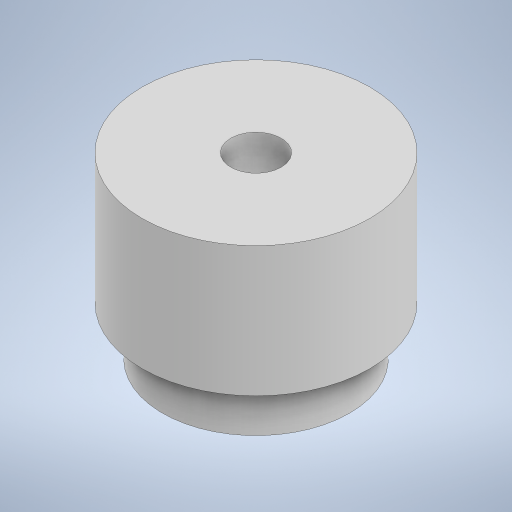
# Autodesk Inventor part: vial
Saved by Autodesk Inventor 2023.1 (Build 271208000, 208)
## iProperties
Created: 2023-05-02
Part Number: vial
Material: Generic
Document SubType Name: Modeling
Designer: dinesh
Density: 1 g/cm^3
Appearance: Default
Author: dinesh
Autodesk Inventor part; units mm, degrees
ref_plane "YZ Plane" through (0, 0, 0) normal (1, 0, 0) x (0, 1, 0)
ref_plane "XZ Plane" through (0, 0, 0) normal (0, 1, 0) x (-1, 0, 0)
ref_plane "XY Plane" through (0, 0, 0) normal (0, 0, 1) x (1, 0, 0)
sketch "Sketch1" plane through (0, 0, 0) normal (0, 0, 1) x (1, 0, 0)
  line L0 (2, 10) -> (14, 10)
  line L1 (14, 10) -> (14, 0)
  line L2 (2, 2) -> (2, 10)
  line L3 (0, 19.5472) -> (0, -22.4151)
  line L4 (14, 0) -> (13, 0) construction
  line L5 (13, 0) -> (13, -6)
  line L6 (13, -6) -> (14, -6)
  line L7 (14, -6) -> (14, 0)
  line L8 (11.5, 0) -> (10.5, 0) construction
  line L9 (10.5, -6) -> (10.5, -6)
  line L10 (10.5, -6) -> (11.5, -6) construction
  line L11 (11.5, -6) -> (11.5, 0)
  line L12 (11.5, -6) -> (11.5, -12)
  line L13 (11.5, -12) -> (11.4, -12)
  line L14 (11.4, -12) -> (10.5, -6)
  arc A0 (2, 2) -> (4, 0) centre (4, 2) ccw
  line L15 (13, 0) -> (11.5, 0)
  line L16 (4.5, 0) -> (4, 0)
  line L17 (-20.0393, 0) -> (13, 0) construction
  line L18 (14, 0) -> (24.5476, 0) construction
  arc A1 (10.5, -6) -> (4.5, 0) centre (4.5, -6) ccw
  point P0 (0, 0)
  point P1 (10.5, -6)
  dimension "d0" = 4
  dimension "d2" = 1
  dimension "d4" = 1
  dimension "d5" = 6
  dimension "d6" = 1.5
  dimension "d7" = 26
  dimension "d9" = 6
  dimension "d10" = 0.1
  dimension "d11" = 2
  dimension "d12" = 10
  dimension "d13" = 6
  dimension "d14" = 6
  constraints: 38 end point, 7 parallel, 5 horizontal, 5 point on line, 5 tangent, 4 collinear, 4 perpendicular, 4 point on circle, 2 centre point, 2 vertical
  measures "d0" diameter of L2 L3
  measures "d2" distance between parallel lines of L5 L7
  measures "d4" distance between parallel lines of L11 L9
  measures "d5" distance between parallel lines of L10 L8
  measures "d6" distance between parallel lines of L5 L11
  measures "d7" diameter of L5 L3
  measures "d9" distance of L10.end L12.end
  measures "d10" distance of L12.end L13.end
  measures "d11" radius of A0
  measures "d12" distance between parallel lines of L16 L0
  measures "d13" radius of A1
  measures "d14" distance between parallel lines of L6 L4
revolve "Revolution1" add sketch "Sketch1" angle 360 about axis through (0, 19.5472, 0) along (0, -1, 0)
sketch "Sketch2" plane through (0, 0, 0) normal (0, 0, 1) x (1, 0, 0)
  line L0 (-4, 0) -> (4, 0) projected
  line L1 (-2, 10) -> (2, 10) projected
  line L2 (0, 10) -> (0, 0) construction
  line L3 (-2, 2) -> (2, 2) construction
  circle A0 centre (0, 2.5) radius 2
  point P0 (1.9365, 2)
  point P1 (-1.9365, 2)
  dimension "d16" = 4
  dimension "d17" = 2.5
  constraints: 2 end point, 1 centre point, 1 midpoint, 1 perpendicular, 1 point on line
  measures "d16" diameter of A0
  measures "d17" distance from line of L0 A0.centre
extrude "Extrusion1" cut sketch "Sketch2" along normal blind 2 and the other way blind 19.5
sketch "Sketch4" plane through (0, 10, 0) normal (0, 1, 0) x (1, 0, 0)
  circle A0 centre (0, 0) radius 3.1
  dimension "d38" = 6.2
  constraints: 1 centre point, 1 coincident
  measures "d38" diameter of A0
extrude "Extrusion3" cut sketch "Sketch4" against normal blind 5
sketch "Sketch3" plane through (0, 10, 0) normal (0, 1, 0) x (1, 0, 0)
  circle A0 centre (-5, 0) radius 0.25
  line L0 (0, 0) -> (-14, 0) construction
  circle A1 centre (0, 0) radius 14 construction
  circle A2 centre (-8, 0) radius 0.25
  circle A3 centre (0, 0) radius 2 construction
  arc A4 (-1.9365, 0.5) -> (-1.9365, -0.5) centre (0, 0) ccw construction
  circle A5 centre (-6.9282, -4) radius 0.25
  circle A6 centre (-4.3301, -2.5) radius 0.25
  circle A7 centre (-4, -6.9282) radius 0.25
  circle A8 centre (-2.5, -4.3301) radius 0.25
  circle A9 centre (0, -8) radius 0.25
  circle A10 centre (0, -5) radius 0.25
  circle A11 centre (4, -6.9282) radius 0.25
  circle A12 centre (2.5, -4.3301) radius 0.25
  circle A13 centre (6.9282, -4) radius 0.25
  circle A14 centre (4.3301, -2.5) radius 0.25
  circle A15 centre (8, 0) radius 0.25
  circle A16 centre (5, 0) radius 0.25
  circle A17 centre (6.9282, 4) radius 0.25
  circle A18 centre (4.3301, 2.5) radius 0.25
  circle A19 centre (4, 6.9282) radius 0.25
  circle A20 centre (2.5, 4.3301) radius 0.25
  circle A21 centre (0, 8) radius 0.25
  circle A22 centre (0, 5) radius 0.25
  circle A23 centre (-4, 6.9282) radius 0.25
  circle A24 centre (-2.5, 4.3301) radius 0.25
  circle A25 centre (-6.9282, 4) radius 0.25
  circle A26 centre (-4.3301, 2.5) radius 0.25
  point P0 (-2, 0)
  point P1 (-2, 0)
  dimension "d22" = 0.5
  dimension "d24" = 0.5
  dimension "d30" = 3
  dimension "d31" = 3
  dimension "d34" = 360
  constraints: 24 centre point, 3 point on line, 2 end point, 2 point on circle, 1 horizontal, 1 horizontal alignment, 50 other
  measures "d22" diameter of A0
  measures "d24" diameter of A2
  measures "d30" distance of A2.centre A0.centre
  measures "d31" distance of point (-2, 0) A0.centre
equation "\"d0\" = t_D"
equation "\"d2\" = w_th"
equation "\"d4\" = w_th"
equation "\"d5\" = w_l"
equation "\"d6\" = lv_th"
equation "\"d7\" = lv_OD"
equation "\"d9\" = w_l"
equation "\"d10\" = tol"
equation "\"d11\" = fillet_D"
equation "\"d12\" = top_th_f"
equation "\"d13\" = 3 * fillet_D"
equation "\"d14\" = w_l"
equation "\"d16\" = t_D"
equation "\"d17\" = 0.5 * w_th + 0.5 * t_D"
equation "\"d18\" = 0.5 * t_D"
equation "\"d19\" = 0.75 * lv_OD"
equation "\"d38\" = cn_D"
equation "\"d39\" = cn_h"
equation "\"d22\" = h_D"
equation "\"d24\" = h_D"
equation "\"d30\" = h_s"
equation "\"d31\" = h_s"
equation "\"tol\" = 0.1"
equation "\"fillet_D\" = 2"
equation "\"w_th\" = 1"
equation "\"w_l\" = 6"
equation "\"t_D\" = 4"
equation "\"t_D_f\" = t_D + w_th"
equation "\"top_th_f\" = t_D_f + cn_h"
equation "\"cn_h\" = 5"
equation "\"lv_OD\" = 26"
equation "\"lv_th\" = 1.5"
equation "\"d3\" = w_l"
equation "\"top_th\" = t_D + w_th"
equation "\"sv_OD\" = 13"
equation "\"sv_th\" = 1.5"
equation "\"b_OD\" = 43.5"
equation "\"b_th\" = 1.5"
equation "\"b_ID\" = 36.5"
equation "\"b_rim_h\" = 5"
equation "\"h_s\" = 3"
equation "\"h_D\" = 5 * tol"
equation "\"d25\" = 2 * d26"
equation "\"cn_D\" = 6.2"
equation "\"d26\" = 0.1"
body "Solid1"
